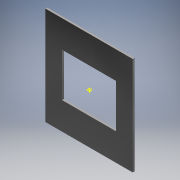
# Autodesk Inventor part: LeftSide
Saved by Autodesk Inventor 2017 (Build 210142000, 142)
## iProperties
Created: 2016-12-12
Part Number: LeftSide
Material: Steel, Mild
Document SubType Name: Sheet Metal
Designer: Robert.Chapman
Density: 7.85 g/cm^3
Sheet Metal Rule: Default
Appearance: Semi-Polished
Mass: 2219.01 g
Surface Area: 1233.55 cm^2
Volume: 282.677 cm^3
Author: Robert.Chapman
Autodesk Inventor part; units mm, degrees
ref_plane "YZ Plane" through (0, 0, 0) normal (1, 0, 0) x (0, 1, 0)
ref_plane "XZ Plane" through (0, 0, 0) normal (0, 1, 0) x (-1, 0, 0)
ref_plane "XY Plane" through (0, 0, 0) normal (0, 0, 1) x (1, 0, 0)
sketch "Sketch1" plane through (0, 0, 0) normal (0, 0, 1) x (1, 0, 0)
  line L0 (112.7125, -127) -> (-112.7125, -127)
  line L1 (-112.7125, -127) -> (-112.7125, 127)
  line L2 (-112.7125, 127) -> (112.7125, 127)
  line L3 (112.7125, 127) -> (112.7125, -127)
  line L4 (112.7125, -127) -> (-112.7125, 127) construction
  line L5 (-112.7125, -127) -> (112.7125, 127) construction
  point P0 (0, 0)
  dimension "d1" = 225.425
  dimension "d2" = 254
  measures "d1" distance of L0.start L0.end
  measures "d2" distance of L2.end L0.start
extrude "Plate1" add sketch "Sketch1" along normal blind 4.7625
sketch "Sketch2" plane through (0, 0, 4.7625) normal (0, 0, 1) x (1, 0, 0)
  line L0 (-69.85, 56.3563) -> (69.85, 56.3563)
  line L1 (69.85, 56.3563) -> (69.85, -56.3563)
  line L2 (69.85, -56.3563) -> (-69.85, -56.3563)
  line L3 (-69.85, -56.3563) -> (-69.85, 56.3563)
  line L4 (-69.85, 56.3563) -> (69.85, -56.3563) construction
  line L5 (69.85, 56.3563) -> (-69.85, -56.3563) construction
  point P0 (0, 0)
  dimension "d3" = 139.7
  dimension "d4" = 112.7125
  constraints: 12 end point, 2 midpoint, 2 parallel, 1 horizontal, 1 perpendicular
  measures "d3" distance of L0.start L0.end
  measures "d4" distance of L0.end L1.end
extrude "Cut1" cut sketch "Sketch2" against normal blind 4.7625
equation "\"d5\" = Thickness"
equation "\"BendRadius\" = Thickness"
equation "\"BendReliefWidth\" = Thickness"
equation "\"BendReliefDepth\" = 0.5 * Thickness"
equation "\"CornerReliefSize\" = 4 * Thickness"
equation "\"MinimumRemnant\" = 2 * Thickness"
equation "\"TransitionRadius\" = BendRadius"
equation "\"JacobiRadiusSize\" = BendRadius"
equation "\"GapSize\" = Thickness"
equation "\"d0\" = BendRadius"
equation "\"Thickness\" = 4.7625"
body "Solid1"
